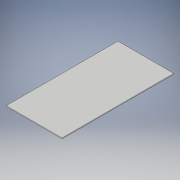
# Autodesk Inventor part: NC.1
Saved by Autodesk Inventor 2019 (Build 230136000, 136)
## iProperties
Created: 2021-11-08
Part Number: NC.1
Material: 一般
Document SubType Name: Sheet Metal
Designer: yuta
Density: 1 g/cm^3
Sheet Metal Rule: Default_mm
Appearance: 既定
Author: yuta
Autodesk Inventor part; units mm, degrees
ref_plane "YZ Plane" through (0, 0, 0) normal (1, 0, 0) x (0, 1, 0)
ref_plane "XZ Plane" through (0, 0, 0) normal (0, 1, 0) x (-1, 0, 0)
ref_plane "XY Plane" through (0, 0, 0) normal (0, 0, 1) x (1, 0, 0)
sketch "スケッチ1" plane through (0, 0, 0) normal (0, 1, 0) x (-1, 0, 0)
  line L0 (6.6919, 11.1938) -> (-193.3081, 11.1938)
  line L1 (-193.3081, 11.1938) -> (-193.3081, -388.8062)
  line L2 (-193.3081, -388.8062) -> (6.6919, -388.8062)
  line L3 (6.6919, -388.8062) -> (6.6919, 11.1938)
  point P0 (0, 0)
  dimension "d0" = 200
  dimension "d1" = 400
  constraints: 8 end point, 2 parallel, 1 horizontal, 1 perpendicular
  measures "d0" distance of L2.end L1.end
  measures "d1" distance of L1.end L0.end
extrude "押し出し1" add sketch "スケッチ1" along normal blind 3
equation "\"BendRadius\" = Thickness"
equation "\"BendReliefWidth\" = Thickness"
equation "\"BendReliefDepth\" = 0.5 * Thickness"
equation "\"CornerReliefSize\" = 4 * Thickness"
equation "\"MinimumRemnant\" = 2 * Thickness"
equation "\"TransitionRadius\" = BendRadius"
equation "\"JacobiRadiusSize\" = BendRadius"
equation "\"GapSize\" = Thickness"
equation "\"Thickness\" = 0.5"
